# Autodesk Inventor part: IC_DIL16-SOIC-16
Saved by Autodesk Inventor 2016 (Build 200138000, 138)
## iProperties
Created: 2016-04-08
Part Number: IC_DIL16-SOIC-16
Material: Generic
Document SubType Name: Modeling
Designer: Paschalis
Density: 1 g/cm^3
Appearance: SOIC-16, IC_DIL16-SOIC-16
Author: Paschalis
Autodesk Inventor part; units mm, degrees
ref_plane "YZ Plane" through (0, 0, 0) normal (1, 0, 0) x (0, 1, 0)
ref_plane "XZ Plane" through (0, 0, 0) normal (0, 1, 0) x (-1, 0, 0)
ref_plane "XY Plane" through (0, 0, 0) normal (0, 0, 1) x (1, 0, 0)
sketch "SOIC-16, IC_DIL16-SOIC-16_81" plane through (0, 0, 0) normal (0, 0, 1) x (1, 0, 0)
  line L0 (-5.7527, 3.1001) -> (5.0162, 3.1001)
  line L1 (5.0162, 3.1001) -> (5.0162, -3.9455)
  line L2 (5.0162, -3.9455) -> (-5.7527, -3.9455)
  line L3 (-5.7527, -3.9455) -> (-5.7527, 3.1001)
  constraints: 8 end point
extrude "Extrusion1" add sketch "SOIC-16, IC_DIL16-SOIC-16_81" along normal blind 1
body "Solid1"
